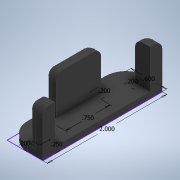
# Autodesk Inventor part: BatteryStopper
Saved by Autodesk Inventor 2020 (Build 240168000, 168)
## iProperties
Created: 2019-06-13
Part Number: BatteryStopper
Material: ABS Plastic
Document SubType Name: Sheet Metal
Designer: amirt
Density: 1.06 g/cm^3
Sheet Metal Rule: Default
Appearance: Dark Gray
Author: amirt
Autodesk Inventor part; units mm, degrees
ref_plane "YZ Plane" through (0, 0, 0) normal (1, 0, 0) x (0, 1, 0)
ref_plane "XZ Plane" through (0, 0, 0) normal (0, 1, 0) x (-1, 0, 0)
ref_plane "XY Plane" through (0, 0, 0) normal (0, 0, 1) x (1, 0, 0)
sketch "Sketch1" plane through (0, 0, 0) normal (0, 1, 0) x (-1, 0, 0)
  line L0 (5.124, 12.8857) -> (-10.116, 12.8857)
  line L1 (-10.116, 12.8857) -> (-10.116, -37.9143)
  line L2 (-10.116, -37.9143) -> (5.124, -37.9143)
  line L3 (5.124, -37.9143) -> (5.124, 12.8857)
  line L4 (-10.116, 12.8857) -> (-3.766, 12.8857)
  line L5 (-3.766, 12.8857) -> (-3.766, 7.8057)
  line L6 (-3.766, 7.8057) -> (-10.116, 7.8057)
  line L7 (-10.116, 7.8057) -> (-10.116, 12.8857)
  line L8 (-10.116, -37.9143) -> (-3.766, -37.9143)
  line L9 (-3.766, -37.9143) -> (-3.766, -32.8343)
  line L10 (-3.766, -32.8343) -> (-10.116, -32.8343)
  line L11 (-10.116, -32.8343) -> (-10.116, -37.9143)
  line L12 (5.124, -2.9893) -> (0.044, -2.9893)
  line L13 (0.044, -2.9893) -> (0.044, -22.0393)
  line L14 (0.044, -22.0393) -> (5.124, -22.0393)
  line L15 (5.124, -22.0393) -> (5.124, -2.9893)
  point P0 (0, 0)
  dimension "d0" = 15.24
  dimension "d1" = 50.8
  dimension "d2" = 6.35
  dimension "d3" = 5.08
  dimension "d4" = 5.08
  dimension "d8" = 5.08
  dimension "d9" = 19.05
  constraints: 32 end point, 8 parallel, 4 horizontal, 4 perpendicular, 2 point on line
  measures "d0" distance of L2.end L1.end
  measures "d1" distance of L1.end L0.end
  measures "d2" distance of L5.end L6.end
  measures "d3" distance of L4.end L5.end
  measures "d4" distance of L9.end L8.end
  measures "d8" distance of L14.end L13.end
  measures "d9" distance of L13.end L12.end
extrude "Extrusion1" add sketch "Sketch1" along normal blind 19.05 contours L5 L6 L1 L0 | L3 L14 L13 L12 | L10 L9 L2 L1
extrude "Extrusion2" add sketch "Sketch1" along normal blind 2.54 contours L3 L12 L13 L14 L2 L9 L10 L1 L6 L5 L0
fillet "Fillet1" radius 8.89 2 edges at (-5.124, 1.27, 12.8857) (-5.124, 1.27, -37.9143)
fillet "Fillet2" radius 3.175 11 edges at (-2.584, 19.05, -2.9893) (-5.124, 19.05, -12.5143) (-5.124, 10.795, -2.9893) (-5.124, 10.795, -22.0393) (-2.584, 19.05, -22.0393) (3.766, 10.795, 12.8857) (3.766, 19.05, 10.3457) (6.941, 19.05, 12.8857) (3.766, 19.05, -35.3743) (6.941, 19.05, -37.9143) (3.766, 10.795, -37.9143)
equation "\"BendRadius\" = Thickness"
equation "\"BendReliefWidth\" = Thickness"
equation "\"BendReliefDepth\" = 0.5 * Thickness"
equation "\"CornerReliefSize\" = 4 * Thickness"
equation "\"MinimumRemnant\" = 2 * Thickness"
equation "\"TransitionRadius\" = BendRadius"
equation "\"JacobiRadiusSize\" = BendRadius"
equation "\"GapSize\" = Thickness"
equation "\"Thickness\" = 3.048"
body "Solid1"
